Autodesk Inventor part; units mm, degrees
(part 2 of 3)
  line L685 (61.8832, -0.1639) -> (61.8305, -0.147) construction
  line L686 (61.936, -0.181) -> (61.8832, -0.1639) construction
  line L687 (61.9887, -0.1981) -> (61.936, -0.181) construction
  line L688 (62.0414, -0.2153) -> (61.9887, -0.1981) construction
  line L689 (62.379, -0.2964) -> (62.0414, -0.2153) construction
  line L690 (62.6505, -0.3259) -> (62.379, -0.2964) construction
  line L691 (62.891, -0.3235) -> (62.6505, -0.3259) construction
  line L692 (63.1221, -0.2997) -> (62.891, -0.3235) construction
  line L693 (63.3379, -0.2543) -> (63.1221, -0.2997) construction
  line L694 (63.5493, -0.1924) -> (63.3379, -0.2543) construction
  line L695 (63.7488, -0.1123) -> (63.5493, -0.1924) construction
  line L696 (63.9434, -0.0172) -> (63.7488, -0.1123) construction
  line L697 (64.1297, 0.0937) -> (63.9434, -0.0172) construction
  line L698 (64.3071, 0.22) -> (64.1297, 0.0937) construction
  line L699 (64.4815, 0.3591) -> (64.3071, 0.22) construction
  line L700 (64.6461, 0.5133) -> (64.4815, 0.3591) construction
  line L701 (64.8026, 0.6817) -> (64.6461, 0.5133) construction
  line L702 (64.9569, 0.8616) -> (64.8026, 0.6817) construction
  line L703 (65.103, 1.0551) -> (64.9569, 0.8616) construction
  line L704 (65.2411, 1.262) -> (65.103, 1.0551) construction
  line L705 (65.3711, 1.4821) -> (65.2411, 1.262) construction
  line L706 (65.4984, 1.7129) -> (65.3711, 1.4821) construction
  line L707 (65.62, 1.9556) -> (65.4984, 1.7129) construction
  line L708 (65.7341, 2.2106) -> (65.62, 1.9556) construction
  line L709 (65.906, 2.5468) -> (65.7341, 2.2106) construction
  line L710 (66.1036, 2.8725) -> (65.906, 2.5468) construction
  line L711 (66.3186, 3.1911) -> (66.1036, 2.8725) construction
  line L712 (66.548, 3.5036) -> (66.3186, 3.1911) construction
  line L713 (66.79, 3.8108) -> (66.548, 3.5036) construction
  line L714 (67.0435, 4.1129) -> (66.79, 3.8108) construction
  line L715 (67.3077, 4.4102) -> (67.0435, 4.1129) construction
  line L716 (67.5819, 4.7028) -> (67.3077, 4.4102) construction
  line L717 (67.8657, 4.991) -> (67.5819, 4.7028) construction
  line L718 (68.1585, 5.2747) -> (67.8657, 4.991) construction
  line L719 (68.4601, 5.5541) -> (68.1585, 5.2747) construction
  line L720 (68.7701, 5.8291) -> (68.4601, 5.5541) construction
  line L721 (69.0883, 6.0998) -> (68.7701, 5.8291) construction
  line L722 (69.4145, 6.3662) -> (69.0883, 6.0998) construction
  line L723 (69.7484, 6.6283) -> (69.4145, 6.3662) construction
  line L724 (70.0899, 6.886) -> (69.7484, 6.6283) construction
  line L725 (70.4388, 7.1393) -> (70.0899, 6.886) construction
  line L726 (70.7949, 7.3883) -> (70.4388, 7.1393) construction
  line L727 (71.1581, 7.6328) -> (70.7949, 7.3883) construction
  line L728 (71.5282, 7.8729) -> (71.1581, 7.6328) construction
  line L729 (71.855, 7.7148) -> (71.5282, 7.8729) construction
  line L730 (72.1807, 7.5544) -> (71.855, 7.7148) construction
  line L731 (72.5051, 7.3915) -> (72.1807, 7.5544) construction
  line L732 (72.8284, 7.2263) -> (72.5051, 7.3915) construction
  line L733 (73.1505, 7.0588) -> (72.8284, 7.2263) construction
  line L734 (73.4713, 6.8889) -> (73.1505, 7.0588) construction
  line L735 (73.7909, 6.7166) -> (73.4713, 6.8889) construction
  line L736 (74.1093, 6.5421) -> (73.7909, 6.7166) construction
  line L737 (74.4263, 6.3652) -> (74.1093, 6.5421) construction
  line L738 (74.7421, 6.186) -> (74.4263, 6.3652) construction
  line L739 (74.7421, 6.186) -> (69.921, -2.2381) construction
  arc A7 (69.921, -2.2381) -> (70.7543, -5.0163) centre (71.6568, -3.2315) ccw construction
  line L740 (70.7543, -5.0163) -> (83.2662, -11.3429) construction
  arc A8 (83.2662, -11.3429) -> (85.055, -11.351) centre (84.1687, -9.5581) ccw construction
  line L741 (85.055, -11.351) -> (116.4248, 4.1568) construction
  arc A9 (119.0371, 3.3744) -> (116.4248, 4.1568) centre (117.3112, 2.3639) ccw construction
  arc A10 (127.7114, -56.0453) -> (119.0371, 3.3744) centre (50, -37.0469) ccw construction
  arc A11 (43.6257, -5.6882) -> (19.6369, -47.1503) centre (50, -37.0469) ccw construction
  arc A12 (19.6369, -47.1503) -> (21.707, -48.5114) centre (21.5346, -46.5189) ccw construction
  line L742 (21.707, -48.5114) -> (35.3323, -47.3323) construction
  arc A13 (35.3323, -47.3323) -> (36.9058, -44.3641) centre (35.1599, -45.3397) ccw construction
  arc A14 (45.1164, -22.8641) -> (36.9058, -44.3641) centre (50, -37.0469) ccw construction
  arc A15 (45.1164, -22.8641) -> (46.4641, -20.9069) centre (44.4652, -20.9731) ccw construction
  line L743 (46.4641, -20.9069) -> (46.023, -7.5819) construction
  arc A16 (46.023, -7.5819) -> (43.6257, -5.6882) centre (44.0241, -7.6481) ccw construction
  arc A17 (57.4364, -24.02) -> (53.9351, -22.5722) centre (50, -37.0469) ccw construction
  arc A18 (57.4364, -24.02) -> (59.3143, -24.076) centre (58.4279, -22.2831) ccw construction
  line L744 (59.3143, -24.076) -> (73.5046, -17.061) construction
  arc A19 (73.5046, -17.061) -> (73.4583, -13.4531) centre (72.6182, -15.2681) ccw construction
  line L745 (73.4583, -13.4531) -> (57.1422, -5.9013) construction
  arc A20 (57.1422, -5.9013) -> (56.7223, -5.7609) centre (56.3021, -7.7163) ccw construction
  arc A21 (56.7223, -5.7609) -> (54.2866, -5.3353) centre (50, -37.0469) ccw construction
  arc A22 (54.2866, -5.3353) -> (52.0197, -7.3834) centre (54.0186, -7.3173) ccw construction
  line L746 (52.0197, -7.3834) -> (52.4608, -20.7084) construction
  arc A23 (52.4608, -20.7084) -> (53.9351, -22.5722) centre (54.4597, -20.6423) ccw construction
  arc A24 (123.9497, -39.7746) -> (120.0838, -13.2926) centre (50, -37.0469) ccw construction
  arc A25 (120.0838, -13.2926) -> (117.3033, -12.1418) centre (118.1896, -13.9346) ccw construction
  line L747 (117.3033, -12.1418) -> (79.5339, -30.8131) construction
  arc A26 (79.5339, -30.8131) -> (80.0834, -34.5775) centre (80.4202, -32.606) ccw construction
  line L748 (80.0834, -34.5775) -> (121.6143, -41.6723) construction
  arc A27 (121.6143, -41.6723) -> (123.9497, -39.7746) centre (121.9511, -39.7009) ccw construction
  circle A28 centre (80.4791, -21.9795) radius 1.2295 construction
  circle A29 centre (83.5145, -42.7723) radius 1.2295 construction
  circle A30 centre (98.3003, -45.2982) radius 1.2295 construction
  circle A31 centre (93.9257, -15.3321) radius 1.2295 construction
  circle A32 centre (50, -37.0469) radius 4 construction
  circle A33 centre (10, -122.0469) radius 1.6 construction
  line L749 (0, -87.0469) -> (20, -87.0469) construction
  line L750 (20, -87.0469) -> (20, -132.0469) construction
  line L751 (0, -132.0469) -> (20, -132.0469) construction
  line L752 (0, -87.0469) -> (0, -132.0469) construction
  circle A34 centre (10, -97.0469) radius 1.6 construction
  circle A35 centre (10, 47.9531) radius 1.6 construction
  line L753 (20, 12.9531) -> (0, 12.9531) construction
  line L754 (0, 57.9531) -> (0, 12.9531) construction
  line L755 (20, 57.9531) -> (0, 57.9531) construction
  line L756 (20, 57.9531) -> (20, 12.9531) construction
  circle A36 centre (10, 22.9531) radius 1.6 construction
  circle A37 centre (50, 24.7653) radius 4 construction
  line L757 (43.5439, 16.1699) -> (43.5808, 16.1423) construction
  line L758 (43.5071, 16.1977) -> (43.5439, 16.1699) construction
  line L759 (43.4704, 16.2256) -> (43.5071, 16.1977) construction
  line L760 (43.4338, 16.2537) -> (43.4704, 16.2256) construction
  line L761 (43.3973, 16.2819) -> (43.4338, 16.2537) construction
  line L762 (43.361, 16.3104) -> (43.3973, 16.2819) construction
  line L763 (43.1086, 16.4778) -> (43.361, 16.3104) construction
  line L764 (42.9044, 16.5756) -> (43.1086, 16.4778) construction
  line L765 (42.6758, 16.6731) -> (42.9044, 16.5756) construction
  line L766 (42.469, 16.7329) -> (42.6758, 16.6731) construction
  line L767 (42.2706, 16.7673) -> (42.469, 16.7329) construction
  line L768 (42.0769, 16.7804) -> (42.2706, 16.7673) construction
  line L769 (41.8782, 16.7823) -> (42.0769, 16.7804) construction
  line L770 (41.6755, 16.7728) -> (41.8782, 16.7823) construction
  line L771 (41.4782, 16.7425) -> (41.6755, 16.7728) construction
  line L772 (41.2858, 16.6918) -> (41.4782, 16.7425) construction
  line L773 (41.0896, 16.6304) -> (41.2858, 16.6918) construction
  line L774 (40.8915, 16.5563) -> (41.0896, 16.6304) construction
  line L775 (40.7008, 16.4595) -> (40.8915, 16.5563) construction
  line L776 (40.5115, 16.3468) -> (40.7008, 16.4595) construction
  line L777 (40.3175, 16.2253) -> (40.5115, 16.3468) construction
  line L778 (40.135, 16.077) -> (40.3175, 16.2253) construction
  line L779 (39.9489, 15.919) -> (40.135, 16.077) construction
  line L780 (39.767, 15.7432) -> (39.9489, 15.919) construction
  line L781 (39.5974, 15.5404) -> (39.767, 15.7432) construction
  line L782 (39.4169, 15.3374) -> (39.5974, 15.5404) construction
  line L783 (39.0835, 15.1378) -> (39.4169, 15.3374) construction
  line L784 (38.7191, 14.9743) -> (39.0835, 15.1378) construction
  line L785 (38.3325, 14.8381) -> (38.7191, 14.9743) construction
  line L786 (37.9275, 14.7263) -> (38.3325, 14.8381) construction
  line L787 (37.5062, 14.6376) -> (37.9275, 14.7263) construction
  line L788 (37.0703, 14.5712) -> (37.5062, 14.6376) construction
  line L789 (36.6212, 14.5267) -> (37.0703, 14.5712) construction
  line L790 (36.1601, 14.504) -> (36.6212, 14.5267) construction
  line L791 (35.6881, 14.503) -> (36.1601, 14.504) construction
  line L792 (35.2063, 14.5239) -> (35.6881, 14.503) construction
  line L793 (34.7154, 14.5666) -> (35.2063, 14.5239) construction
  line L794 (34.2166, 14.6313) -> (34.7154, 14.5666) construction
  line L795 (33.7106, 14.7183) -> (34.2166, 14.6313) construction
  line L796 (33.1984, 14.8275) -> (33.7106, 14.7183) construction
  line L797 (32.6809, 14.9593) -> (33.1984, 14.8275) construction
  line L798 (32.1588, 15.1139) -> (32.6809, 14.9593) construction
  line L799 (31.6332, 15.2912) -> (32.1588, 15.1139) construction
  line L800 (31.1048, 15.4916) -> (31.6332, 15.2912) construction
  line L801 (30.5745, 15.7152) -> (31.1048, 15.4916) construction
  line L802 (30.0432, 15.9621) -> (30.5745, 15.7152) construction
  line L803 (30.0213, 16.0118) -> (30.0432, 15.9621) construction
  line L804 (29.9996, 16.0616) -> (30.0213, 16.0118) construction
  line L805 (29.978, 16.1115) -> (29.9996, 16.0616) construction
  line L806 (29.9565, 16.1614) -> (29.978, 16.1115) construction
  line L807 (29.9351, 16.2113) -> (29.9565, 16.1614) construction
  line L808 (29.9138, 16.2613) -> (29.9351, 16.2113) construction
  line L809 (29.8927, 16.3114) -> (29.9138, 16.2613) construction
  line L810 (29.8717, 16.3615) -> (29.8927, 16.3114) construction
  line L811 (29.8509, 16.4117) -> (29.8717, 16.3615) construction
  line L812 (29.8301, 16.4619) -> (29.8509, 16.4117) construction
  line L813 (30.0199, 17.0162) -> (29.8301, 16.4619) construction
  line L814 (30.2257, 17.5536) -> (30.0199, 17.0162) construction
  line L815 (30.447, 18.0736) -> (30.2257, 17.5536) construction
  line L816 (30.683, 18.5756) -> (30.447, 18.0736) construction
  line L817 (30.933, 19.0593) -> (30.683, 18.5756) construction
  line L818 (31.1963, 19.524) -> (30.933, 19.0593) construction
  line L819 (31.4721, 19.9692) -> (31.1963, 19.524) construction
  line L820 (31.7597, 20.3944) -> (31.4721, 19.9692) construction
  line L821 (32.0584, 20.7992) -> (31.7597, 20.3944) construction
  line L822 (32.3674, 21.1829) -> (32.0584, 20.7992) construction
  line L823 (32.6861, 21.545) -> (32.3674, 21.1829) construction
  line L824 (33.0136, 21.8849) -> (32.6861, 21.545) construction
  line L825 (33.3492, 22.2018) -> (33.0136, 21.8849) construction
  line L826 (33.6922, 22.495) -> (33.3492, 22.2018) construction
  line L827 (34.0419, 22.7635) -> (33.6922, 22.495) construction
  line L828 (34.3977, 23.0061) -> (34.0419, 22.7635) construction
  line L829 (34.7588, 23.2209) -> (34.3977, 23.0061) construction
  line L830 (35.1247, 23.4055) -> (34.7588, 23.2209) construction
  line L831 (35.495, 23.5553) -> (35.1247, 23.4055) construction
  line L832 (35.8699, 23.6576) -> (35.495, 23.5553) construction
  line L833 (36.1413, 23.6472) -> (35.8699, 23.6576) construction
  line L834 (36.405, 23.6292) -> (36.1413, 23.6472) construction
  line L835 (36.6579, 23.6387) -> (36.405, 23.6292) construction
  line L836 (36.9007, 23.6635) -> (36.6579, 23.6387) construction
  line L837 (37.1341, 23.6926) -> (36.9007, 23.6635) construction
  line L838 (37.3561, 23.7483) -> (37.1341, 23.6926) construction
  line L839 (37.5685, 23.8069) -> (37.3561, 23.7483) construction
  line L840 (37.7703, 23.8775) -> (37.5685, 23.8069) construction
  line L841 (37.9609, 23.9691) -> (37.7703, 23.8775) construction
  line L842 (38.1412, 24.0682) -> (37.9609, 23.9691) construction
  line L843 (38.3109, 24.1719) -> (38.1412, 24.0682) construction
  line L844 (38.4694, 24.2932) -> (38.3109, 24.1719) construction
  line L845 (38.6166, 24.433) -> (38.4694, 24.2932) construction
  line L846 (38.7528, 24.5776) -> (38.6166, 24.433) construction
  line L847 (38.8775, 24.7264) -> (38.7528, 24.5776) construction
  line L848 (38.9901, 24.8934) -> (38.8775, 24.7264) construction
  line L849 (39.0901, 25.084) -> (38.9901, 24.8934) construction
  line L850 (39.178, 25.3165) -> (39.0901, 25.084) construction
  line L851 (39.2489, 25.5315) -> (39.178, 25.3165) construction
  line L852 (39.3028, 25.8295) -> (39.2489, 25.5315) construction
  line L853 (39.3075, 25.8754) -> (39.3028, 25.8295) construction
  line L854 (39.3123, 25.9213) -> (39.3075, 25.8754) construction
  line L855 (39.3174, 25.9671) -> (39.3123, 25.9213) construction
  line L856 (39.3226, 26.013) -> (39.3174, 25.9671) construction
  line L857 (39.3281, 26.0588) -> (39.3226, 26.013) construction
  line L858 (39.3337, 26.1045) -> (39.3281, 26.0588) construction
  line L859 (39.3396, 26.1503) -> (39.3337, 26.1045) construction
  line L860 (39.3456, 26.196) -> (39.3396, 26.1503) construction
  line L861 (39.3519, 26.2417) -> (39.3456, 26.196) construction
  line L862 (39.3583, 26.2874) -> (39.3519, 26.2417) construction
  line L863 (39.3772, 26.5897) -> (39.3583, 26.2874) construction
  line L864 (39.3597, 26.8154) -> (39.3772, 26.5897) construction
  line L865 (39.3299, 27.0621) -> (39.3597, 26.8154) construction
  line L866 (39.2783, 27.2712) -> (39.3299, 27.0621) construction
  line L867 (39.2089, 27.4602) -> (39.2783, 27.2712) construction
  line L868 (39.1234, 27.6345) -> (39.2089, 27.4602) construction
  line L869 (39.0256, 27.8074) -> (39.1234, 27.6345) construction
  line L870 (38.9161, 27.9783) -> (39.0256, 27.8074) construction
  line L871 (38.7911, 28.134) -> (38.9161, 27.9783) construction
  line L872 (38.6511, 28.2752) -> (38.7911, 28.134) construction
  line L873 (38.4997, 28.4145) -> (38.6511, 28.2752) construction
  line L874 (38.3366, 28.549) -> (38.4997, 28.4145) construction
  line L875 (38.1574, 28.6658) -> (38.3366, 28.549) construction
  line L876 (37.9652, 28.7734) -> (38.1574, 28.6658) construction
  line L877 (37.7629, 28.8805) -> (37.9652, 28.7734) construction
  line L878 (37.5432, 28.9645) -> (37.7629, 28.8805) construction
  line L879 (37.3134, 29.0466) -> (37.5432, 28.9645) construction
  line L880 (37.0701, 29.1163) -> (37.3134, 29.0466) construction
  line L881 (36.8097, 29.1618) -> (37.0701, 29.1163) construction
  line L882 (36.5437, 29.2166) -> (36.8097, 29.1618) construction
  line L883 (36.2041, 29.4055) -> (36.5437, 29.2166) construction
  line L884 (35.8803, 29.6394) -> (36.2041, 29.4055) construction
  line L885 (35.569, 29.906) -> (35.8803, 29.6394) construction
  line L886 (35.2697, 30.2009) -> (35.569, 29.906) construction
  line L887 (34.9822, 30.5214) -> (35.2697, 30.2009) construction
  line L888 (34.7068, 30.8657) -> (34.9822, 30.5214) construction
  line L889 (34.4437, 31.2324) -> (34.7068, 30.8657) construction
  line L890 (34.1935, 31.6203) -> (34.4437, 31.2324) construction
  line L891 (33.9567, 32.0286) -> (34.1935, 31.6203) construction
  line L892 (33.7338, 32.4563) -> (33.9567, 32.0286) construction
  line L893 (33.5254, 32.9028) -> (33.7338, 32.4563) construction
  line L894 (33.332, 33.3671) -> (33.5254, 32.9028) construction
  line L895 (33.1543, 33.8488) -> (33.332, 33.3671) construction
  line L896 (32.9929, 34.347) -> (33.1543, 33.8488) construction
  line L897 (32.8482, 34.8611) -> (32.9929, 34.347) construction
  line L898 (32.721, 35.3905) -> (32.8482, 34.8611) construction
  line L899 (32.6118, 35.9344) -> (32.721, 35.3905) construction
  line L900 (32.5212, 36.4922) -> (32.6118, 35.9344) construction
  line L901 (32.4496, 37.0632) -> (32.5212, 36.4922) construction
  line L902 (32.3978, 37.6468) -> (32.4496, 37.0632) construction
  line L903 (32.4299, 37.6906) -> (32.3978, 37.6468) construction
  line L904 (32.4622, 37.7343) -> (32.4299, 37.6906) construction
  line L905 (32.4945, 37.778) -> (32.4622, 37.7343) construction
  line L906 (32.527, 37.8215) -> (32.4945, 37.778) construction
  line L907 (32.5596, 37.865) -> (32.527, 37.8215) construction
  line L908 (32.5923, 37.9084) -> (32.5596, 37.865) construction
  line L909 (32.6251, 37.9518) -> (32.5923, 37.9084) construction
  line L910 (32.658, 37.995) -> (32.6251, 37.9518) construction
  line L911 (32.691, 38.0382) -> (32.658, 37.995) construction
  line L912 (32.7241, 38.0812) -> (32.691, 38.0382) construction
  line L913 (33.299, 38.194) -> (32.7241, 38.0812) construction
  line L914 (33.8673, 38.2844) -> (33.299, 38.194) construction
  line L915 (34.4283, 38.3528) -> (33.8673, 38.2844) construction
  line L916 (34.9811, 38.3995) -> (34.4283, 38.3528) construction
  line L917 (35.525, 38.4248) -> (34.9811, 38.3995) construction
  line L918 (36.059, 38.4291) -> (35.525, 38.4248) construction
  line L919 (36.5825, 38.4129) -> (36.059, 38.4291) construction
  line L920 (37.0946, 38.3764) -> (36.5825, 38.4129) construction
  line L921 (37.5944, 38.3201) -> (37.0946, 38.3764) construction
  line L922 (38.0813, 38.2443) -> (37.5944, 38.3201) construction
  line L923 (38.5542, 38.1494) -> (38.0813, 38.2443) construction
  line L924 (39.0122, 38.0358) -> (38.5542, 38.1494) construction
  line L925 (39.4545, 37.9036) -> (39.0122, 38.0358) construction
  line L926 (39.88, 37.7531) -> (39.4545, 37.9036) construction
  line L927 (40.2874, 37.5845) -> (39.88, 37.7531) construction
  line L928 (40.6753, 37.3977) -> (40.2874, 37.5845) construction
  line L929 (41.042, 37.1924) -> (40.6753, 37.3977) construction
  line L930 (41.3848, 36.9678) -> (41.042, 37.1924) construction
  line L931 (41.6996, 36.722) -> (41.3848, 36.9678) construction
  line L932 (41.9756, 36.4484) -> (41.6996, 36.722) construction
  line L933 (42.1024, 36.2082) -> (41.9756, 36.4484) construction
  line L934 (42.2186, 35.9708) -> (42.1024, 36.2082) construction
  line L935 (42.3533, 35.7566) -> (42.2186, 35.9708) construction
  line L936 (42.4962, 35.5588) -> (42.3533, 35.7566) construction
  line L937 (42.6381, 35.3711) -> (42.4962, 35.5588) construction
  line L938 (42.7974, 35.2068) -> (42.6381, 35.3711) construction
  line L939 (42.9543, 35.0521) -> (42.7974, 35.2068) construction
  line L940 (43.1163, 34.9126) -> (42.9543, 35.0521) construction
  line L941 (43.291, 34.7933) -> (43.1163, 34.9126) construction
  line L942 (43.4669, 34.6868) -> (43.291, 34.7933) construction
  line L943 (43.6416, 34.5916) -> (43.4669, 34.6868) construction
  line L944 (43.8259, 34.515) -> (43.6416, 34.5916) construction
  line L945 (44.0205, 34.4574) -> (43.8259, 34.515) construction
  line L946 (44.2138, 34.4117) -> (44.0205, 34.4574) construction
  line L947 (44.4051, 34.3782) -> (44.2138, 34.4117) construction
  line L948 (44.606, 34.3642) -> (44.4051, 34.3782) construction
  line L949 (44.8211, 34.3729) -> (44.606, 34.3642) construction
  line L950 (45.0664, 34.413) -> (44.8211, 34.3729) construction
  line L951 (45.288, 34.4591) -> (45.0664, 34.413) construction
  line L952 (45.5731, 34.5615) -> (45.288, 34.4591) construction
  line L953 (45.6151, 34.5804) -> (45.5731, 34.5615) construction
  line L954 (45.6573, 34.5991) -> (45.6151, 34.5804) construction
  line L955 (45.6995, 34.6176) -> (45.6573, 34.5991) construction
  line L956 (45.7418, 34.636) -> (45.6995, 34.6176) construction
  line L957 (45.7842, 34.6542) -> (45.7418, 34.636) construction
  line L958 (45.8267, 34.6722) -> (45.7842, 34.6542) construction
  line L959 (45.8692, 34.69) -> (45.8267, 34.6722) construction
  line L960 (45.9119, 34.7076) -> (45.8692, 34.69) construction
  line L961 (45.9546, 34.725) -> (45.9119, 34.7076) construction
  line L962 (45.9973, 34.7423) -> (45.9546, 34.725) construction
  line L963 (46.2685, 34.8771) -> (45.9973, 34.7423) construction
  line L964 (46.4553, 35.0051) -> (46.2685, 34.8771) construction
  line L965 (46.6541, 35.1543) -> (46.4553, 35.0051) construction
  line L966 (46.8093, 35.3035) -> (46.6541, 35.1543) construction
  line L967 (46.9383, 35.4581) -> (46.8093, 35.3035) construction
  line L968 (47.0465, 35.6193) -> (46.9383, 35.4581) construction
  line L969 (47.1474, 35.7905) -> (47.0465, 35.6193) construction
  line L970 (47.2406, 35.9708) -> (47.1474, 35.7905) construction
  line L971 (47.3129, 36.1568) -> (47.2406, 35.9708) construction
  line L972 (47.3652, 36.3487) -> (47.3129, 36.1568) construction
  line L973 (47.4102, 36.5494) -> (47.3652, 36.3487) construction
  line L974 (47.4451, 36.758) -> (47.4102, 36.5494) construction
  line L975 (47.4566, 36.9715) -> (47.4451, 36.758) construction
  line L976 (47.4537, 37.1918) -> (47.4566, 36.9715) construction
  line L977 (47.4454, 37.4206) -> (47.4537, 37.1918) construction
  line L978 (47.4082, 37.6528) -> (47.4454, 37.4206) construction
  line L979 (47.3644, 37.8929) -> (47.4082, 37.6528) construction
  line L980 (47.3031, 38.1384) -> (47.3644, 37.8929) construction
  line L981 (47.2124, 38.3867) -> (47.3031, 38.1384) construction
  line L982 (47.1268, 38.6444) -> (47.2124, 38.3867) construction
  line L983 (47.1206, 39.033) -> (47.1268, 38.6444) construction
  line L984 (47.1612, 39.4304) -> (47.1206, 39.033) construction
  line L985 (47.2365, 39.8332) -> (47.1612, 39.4304) construction
  line L986 (47.3422, 40.2399) -> (47.2365, 39.8332) construction
  line L987 (47.4761, 40.6491) -> (47.3422, 40.2399) construction
  line L988 (47.6365, 41.0598) -> (47.4761, 40.6491) construction
  line L989 (47.8225, 41.471) -> (47.6365, 41.0598) construction
  line L990 (48.0334, 41.8816) -> (47.8225, 41.471) construction
  line L991 (48.2686, 42.2908) -> (48.0334, 41.8816) construction
  line L992 (48.5275, 42.6977) -> (48.2686, 42.2908) construction
  line L993 (48.8099, 43.1015) -> (48.5275, 42.6977) construction
  line L994 (49.1154, 43.5011) -> (48.8099, 43.1015) construction
  line L995 (49.4437, 43.8958) -> (49.1154, 43.5011) construction
  line L996 (49.7944, 44.2848) -> (49.4437, 43.8958) construction
  line L997 (50.1674, 44.6671) -> (49.7944, 44.2848) construction
  line L998 (50.5622, 45.0419) -> (50.1674, 44.6671) construction
  line L999 (50.9787, 45.4085) -> (50.5622, 45.0419) construction
  line L1000 (51.4164, 45.7659) -> (50.9787, 45.4085) construction
  line L1001 (51.8752, 46.1133) -> (51.4164, 45.7659) construction
  line L1002 (52.3546, 46.45) -> (51.8752, 46.1133) construction
  line L1003 (52.4086, 46.4441) -> (52.3546, 46.45) construction
  line L1004 (52.4626, 46.438) -> (52.4086, 46.4441) construction
  line L1005 (52.5166, 46.4318) -> (52.4626, 46.438) construction
  line L1006 (52.5705, 46.4255) -> (52.5166, 46.4318) construction
  line L1007 (52.6245, 46.419) -> (52.5705, 46.4255) construction
  line L1008 (52.6784, 46.4124) -> (52.6245, 46.419) construction
  line L1009 (52.7324, 46.4056) -> (52.6784, 46.4124) construction
  line L1010 (52.7863, 46.3988) -> (52.7324, 46.4056) construction
  line L1011 (52.8401, 46.3918) -> (52.7863, 46.3988) construction
  line L1012 (52.894, 46.3846) -> (52.8401, 46.3918) construction
  line L1013 (53.2791, 45.9432) -> (52.894, 46.3846) construction
  line L1014 (53.6416, 45.4962) -> (53.2791, 45.9432) construction
  line L1015 (53.9813, 45.0445) -> (53.6416, 45.4962) construction
  line L1016 (54.2981, 44.5891) -> (53.9813, 45.0445) construction
  line L1017 (54.592, 44.1308) -> (54.2981, 44.5891) construction
  line L1018 (54.8628, 43.6705) -> (54.592, 44.1308) construction
  line L1019 (55.1104, 43.209) -> (54.8628, 43.6705) construction
  line L1020 (55.3349, 42.7473) -> (55.1104, 43.209) construction
  line L1021 (55.5361, 42.2862) -> (55.3349, 42.7473) construction
  line L1022 (55.7138, 41.8267) -> (55.5361, 42.2862) construction
  line L1023 (55.8681, 41.3697) -> (55.7138, 41.8267) construction
  line L1024 (55.9987, 40.9162) -> (55.8681, 41.3697) construction
  line L1025 (56.1054, 40.4671) -> (55.9987, 40.9162) construction
  line L1026 (56.1878, 40.0234) -> (56.1054, 40.4671) construction
  line L1027 (56.2455, 39.5863) -> (56.1878, 40.0234) construction
  line L1028 (56.2776, 39.1569) -> (56.2455, 39.5863) construction
  line L1029 (56.2832, 38.7367) -> (56.2776, 39.1569) construction
  line L1030 (56.26, 38.3276) -> (56.2832, 38.7367) construction
  line L1031 (56.2046, 37.932) -> (56.26, 38.3276) construction
  line L1032 (56.1057, 37.5562) -> (56.2046, 37.932) construction
  line L1033 (55.961, 37.3263) -> (56.1057, 37.5562) construction
  line L1034 (55.8136, 37.1069) -> (55.961, 37.3263) construction
  line L1035 (55.6954, 36.8832) -> (55.8136, 37.1069) construction
  line L1036 (55.5955, 36.6605) -> (55.6954, 36.8832) construction
  line L1037 (55.504, 36.4438) -> (55.5955, 36.6605) construction
  line L1038 (55.4413, 36.2237) -> (55.504, 36.4438) construction
  line L1039 (55.3858, 36.0105) -> (55.4413, 36.2237) construction
  line L1040 (55.3459, 35.8004) -> (55.3858, 36.0105) construction
  line L1041 (55.33, 35.5895) -> (55.3459, 35.8004) construction
  line L1042 (55.3257, 35.3839) -> (55.33, 35.5895) construction
  line L1043 (55.3307, 35.185) -> (55.3257, 35.3839) construction
  line L1044 (55.3565, 34.9871) -> (55.3307, 35.185) construction
  line L1045 (55.4039, 34.7897) -> (55.3565, 34.9871) construction
  line L1046 (55.461, 34.5995) -> (55.4039, 34.7897) construction
  line L1047 (55.5276, 34.4171) -> (55.461, 34.5995) construction
  line L1048 (55.6159, 34.2361) -> (55.5276, 34.4171) construction
  line L1049 (55.731, 34.0541) -> (55.6159, 34.2361) construction
  line L1050 (55.8883, 33.8618) -> (55.731, 34.0541) construction
  line L1051 (56.0391, 33.6929) -> (55.8883, 33.8618) construction
  line L1052 (56.2703, 33.4972) -> (56.0391, 33.6929) construction
  line L1053 (56.3077, 33.4702) -> (56.2703, 33.4972) construction
  line L1054 (56.345, 33.4431) -> (56.3077, 33.4702) construction
  line L1055 (56.3821, 33.4158) -> (56.345, 33.4431) construction
  line L1056 (56.4192, 33.3883) -> (56.3821, 33.4158) construction
  line L1057 (56.4561, 33.3607) -> (56.4192, 33.3883) construction
  line L1058 (56.4929, 33.3329) -> (56.4561, 33.3607) construction
  line L1059 (56.5296, 33.305) -> (56.4929, 33.3329) construction
  line L1060 (56.5662, 33.2769) -> (56.5296, 33.305) construction
  line L1061 (56.6027, 33.2486) -> (56.5662, 33.2769) construction
  line L1062 (56.639, 33.2202) -> (56.6027, 33.2486) construction
  line L1063 (56.8914, 33.0528) -> (56.639, 33.2202) construction
  line L1064 (57.0956, 32.955) -> (56.8914, 33.0528) construction
  line L1065 (57.3242, 32.8575) -> (57.0956, 32.955) construction
  line L1066 (57.531, 32.7977) -> (57.3242, 32.8575) construction
  line L1067 (57.7294, 32.7632) -> (57.531, 32.7977) construction
  line L1068 (57.9231, 32.7501) -> (57.7294, 32.7632) construction
  line L1069 (58.1218, 32.7483) -> (57.9231, 32.7501) construction
  line L1070 (58.3245, 32.7578) -> (58.1218, 32.7483) construction
  line L1071 (58.5218, 32.7881) -> (58.3245, 32.7578) construction
  line L1072 (58.7142, 32.8388) -> (58.5218, 32.7881) construction
  line L1073 (58.9104, 32.9002) -> (58.7142, 32.8388) construction
  line L1074 (59.1085, 32.9742) -> (58.9104, 32.9002) construction
  line L1075 (59.2992, 33.071) -> (59.1085, 32.9742) construction
  line L1076 (59.4885, 33.1837) -> (59.2992, 33.071) construction
  line L1077 (59.6825, 33.3053) -> (59.4885, 33.1837) construction
  line L1078 (59.865, 33.4536) -> (59.6825, 33.3053) construction
  line L1079 (60.0511, 33.6116) -> (59.865, 33.4536) construction
  line L1080 (60.233, 33.7874) -> (60.0511, 33.6116) construction
  line L1081 (60.4026, 33.9901) -> (60.233, 33.7874) construction
  line L1082 (60.5831, 34.1932) -> (60.4026, 33.9901) construction
  line L1083 (60.9165, 34.3928) -> (60.5831, 34.1932) construction
  line L1084 (61.2809, 34.5563) -> (60.9165, 34.3928) construction
  line L1085 (61.6675, 34.6925) -> (61.2809, 34.5563) construction
  line L1086 (62.0725, 34.8043) -> (61.6675, 34.6925) construction
  line L1087 (62.4938, 34.893) -> (62.0725, 34.8043) construction
  line L1088 (62.9297, 34.9594) -> (62.4938, 34.893) construction
  line L1089 (63.3788, 35.0039) -> (62.9297, 34.9594) construction
  line L1090 (63.8399, 35.0266) -> (63.3788, 35.0039) construction
  line L1091 (64.3119, 35.0275) -> (63.8399, 35.0266) construction
  line L1092 (64.7937, 35.0067) -> (64.3119, 35.0275) construction
  line L1093 (65.2846, 34.964) -> (64.7937, 35.0067) construction
  line L1094 (65.7834, 34.8992) -> (65.2846, 34.964) construction
  line L1095 (66.2894, 34.8123) -> (65.7834, 34.8992) construction
  line L1096 (66.8016, 34.703) -> (66.2894, 34.8123) construction
  line L1097 (67.3191, 34.5712) -> (66.8016, 34.703) construction
  line L1098 (67.8412, 34.4167) -> (67.3191, 34.5712) construction
  line L1099 (68.3668, 34.2393) -> (67.8412, 34.4167) construction
  line L1100 (68.8952, 34.0389) -> (68.3668, 34.2393) construction
  line L1101 (69.4255, 33.8154) -> (68.8952, 34.0389) construction
  line L1102 (69.9568, 33.5685) -> (69.4255, 33.8154) construction
  line L1103 (69.9787, 33.5188) -> (69.9568, 33.5685) construction
  line L1104 (70.0004, 33.469) -> (69.9787, 33.5188) construction
  line L1105 (70.022, 33.4191) -> (70.0004, 33.469) construction
  line L1106 (70.0435, 33.3692) -> (70.022, 33.4191) construction
  line L1107 (70.0649, 33.3193) -> (70.0435, 33.3692) construction
  line L1108 (70.0862, 33.2692) -> (70.0649, 33.3193) construction
  line L1109 (70.1073, 33.2192) -> (70.0862, 33.2692) construction
  line L1110 (70.1283, 33.1691) -> (70.1073, 33.2192) construction
  line L1111 (70.1491, 33.1189) -> (70.1283, 33.1691) construction
  line L1112 (70.1699, 33.0687) -> (70.1491, 33.1189) construction
  line L1113 (69.9801, 32.5144) -> (70.1699, 33.0687) construction
  line L1114 (69.7743, 31.977) -> (69.9801, 32.5144) construction
  line L1115 (69.553, 31.457) -> (69.7743, 31.977) construction
  line L1116 (69.317, 30.9549) -> (69.553, 31.457) construction
  line L1117 (69.067, 30.4713) -> (69.317, 30.9549) construction
  line L1118 (68.8037, 30.0066) -> (69.067, 30.4713) construction
  line L1119 (68.5279, 29.5614) -> (68.8037, 30.0066) construction
  line L1120 (68.2403, 29.1361) -> (68.5279, 29.5614) construction
  line L1121 (67.9416, 28.7314) -> (68.2403, 29.1361) construction
  line L1122 (67.6326, 28.3477) -> (67.9416, 28.7314) construction
  line L1123 (67.3139, 27.9856) -> (67.6326, 28.3477) construction
  line L1124 (66.9864, 27.6457) -> (67.3139, 27.9856) construction
  line L1125 (66.6508, 27.3288) -> (66.9864, 27.6457) construction
  line L1126 (66.3078, 27.0356) -> (66.6508, 27.3288) construction
  line L1127 (65.9581, 26.767) -> (66.3078, 27.0356) construction
  line L1128 (65.6023, 26.5245) -> (65.9581, 26.767) construction
  line L1129 (65.2412, 26.3096) -> (65.6023, 26.5245) construction
  line L1130 (64.8753, 26.1251) -> (65.2412, 26.3096) construction
  line L1131 (64.505, 25.9753) -> (64.8753, 26.1251) construction
  line L1132 (64.1301, 25.873) -> (64.505, 25.9753) construction
  line L1133 (63.8587, 25.8834) -> (64.1301, 25.873) construction
  line L1134 (63.595, 25.9014) -> (63.8587, 25.8834) construction
  line L1135 (63.3421, 25.8918) -> (63.595, 25.9014) construction
  line L1136 (63.0993, 25.867) -> (63.3421, 25.8918) construction
  line L1137 (62.8659, 25.838) -> (63.0993, 25.867) construction
  line L1138 (62.6439, 25.7822) -> (62.8659, 25.838) construction
  line L1139 (62.4315, 25.7237) -> (62.6439, 25.7822) construction
  line L1140 (62.2297, 25.6531) -> (62.4315, 25.7237) construction
  line L1141 (62.0391, 25.5615) -> (62.2297, 25.6531) construction
  line L1142 (61.8588, 25.4624) -> (62.0391, 25.5615) construction
  line L1143 (61.6891, 25.3587) -> (61.8588, 25.4624) construction
  line L1144 (61.5306, 25.2373) -> (61.6891, 25.3587) construction
  line L1145 (61.3834, 25.0976) -> (61.5306, 25.2373) construction
  line L1146 (61.2472, 24.953) -> (61.3834, 25.0976) construction
  line L1147 (61.1225, 24.8042) -> (61.2472, 24.953) construction
  line L1148 (61.0099, 24.6372) -> (61.1225, 24.8042) construction
  line L1149 (60.9099, 24.4466) -> (61.0099, 24.6372) construction
  line L1150 (60.822, 24.2141) -> (60.9099, 24.4466) construction
  line L1151 (60.7511, 23.9991) -> (60.822, 24.2141) construction
  line L1152 (60.6972, 23.701) -> (60.7511, 23.9991) construction
  line L1153 (60.6925, 23.6551) -> (60.6972, 23.701) construction
  line L1154 (60.6877, 23.6093) -> (60.6925, 23.6551) construction
  line L1155 (60.6826, 23.5634) -> (60.6877, 23.6093) construction
  line L1156 (60.6774, 23.5176) -> (60.6826, 23.5634) construction
  line L1157 (60.6719, 23.4718) -> (60.6774, 23.5176) construction
  line L1158 (60.6663, 23.426) -> (60.6719, 23.4718) construction
  line L1159 (60.6604, 23.3803) -> (60.6663, 23.426) construction
  line L1160 (60.6544, 23.3346) -> (60.6604, 23.3803) construction
  line L1161 (60.6481, 23.2889) -> (60.6544, 23.3346) construction
  line L1162 (60.6417, 23.2432) -> (60.6481, 23.2889) construction
  line L1163 (60.6228, 22.9409) -> (60.6417, 23.2432) construction
  line L1164 (60.6403, 22.7152) -> (60.6228, 22.9409) construction
  line L1165 (60.6701, 22.4685) -> (60.6403, 22.7152) construction
  line L1166 (60.7217, 22.2594) -> (60.6701, 22.4685) construction
  line L1167 (60.7911, 22.0704) -> (60.7217, 22.2594) construction
  line L1168 (60.8766, 21.8961) -> (60.7911, 22.0704) construction
  line L1169 (60.9744, 21.7231) -> (60.8766, 21.8961) construction
  line L1170 (61.0839, 21.5523) -> (60.9744, 21.7231) construction
  line L1171 (61.2089, 21.3966) -> (61.0839, 21.5523) construction
  line L1172 (61.3489, 21.2553) -> (61.2089, 21.3966) construction
  line L1173 (61.5003, 21.1161) -> (61.3489, 21.2553) construction
  line L1174 (61.6634, 20.9815) -> (61.5003, 21.1161) construction
  line L1175 (61.8426, 20.8648) -> (61.6634, 20.9815) construction
  line L1176 (62.0348, 20.7572) -> (61.8426, 20.8648) construction
  line L1177 (62.2371, 20.65) -> (62.0348, 20.7572) construction
  line L1178 (62.4568, 20.5661) -> (62.2371, 20.65) construction
  line L1179 (62.6866, 20.484) -> (62.4568, 20.5661) construction
  line L1180 (62.9299, 20.4143) -> (62.6866, 20.484) construction
  line L1181 (63.1903, 20.3688) -> (62.9299, 20.4143) construction
  line L1182 (63.4563, 20.314) -> (63.1903, 20.3688) construction
  line L1183 (63.7959, 20.1251) -> (63.4563, 20.314) construction
  line L1184 (64.1197, 19.8912) -> (63.7959, 20.1251) construction
  line L1185 (64.431, 19.6246) -> (64.1197, 19.8912) construction
  line L1186 (64.7303, 19.3297) -> (64.431, 19.6246) construction
  line L1187 (65.0178, 19.0092) -> (64.7303, 19.3297) construction
  line L1188 (65.2932, 18.6649) -> (65.0178, 19.0092) construction
  line L1189 (65.5563, 18.2982) -> (65.2932, 18.6649) construction
  line L1190 (65.8065, 17.9102) -> (65.5563, 18.2982) construction
  line L1191 (66.0433, 17.502) -> (65.8065, 17.9102) construction
  line L1192 (66.2662, 17.0742) -> (66.0433, 17.502) construction
  line L1193 (66.4746, 16.6278) -> (66.2662, 17.0742) construction
  line L1194 (66.668, 16.1634) -> (66.4746, 16.6278) construction
  line L1195 (66.8457, 15.6818) -> (66.668, 16.1634) construction
  line L1196 (67.0071, 15.1836) -> (66.8457, 15.6818) construction
  line L1197 (67.1518, 14.6694) -> (67.0071, 15.1836) construction
  line L1198 (67.279, 14.1401) -> (67.1518, 14.6694) construction
  line L1199 (67.3882, 13.5962) -> (67.279, 14.1401) construction
  line L1200 (67.4788, 13.0383) -> (67.3882, 13.5962) construction
  line L1201 (67.5504, 12.4673) -> (67.4788, 13.0383) construction
  line L1202 (67.6022, 11.8838) -> (67.5504, 12.4673) construction
  line L1203 (67.5701, 11.84) -> (67.6022, 11.8838) construction
  line L1204 (67.5378, 11.7963) -> (67.5701, 11.84) construction
  line L1205 (67.5055, 11.7526) -> (67.5378, 11.7963) construction
  line L1206 (67.473, 11.709) -> (67.5055, 11.7526) construction
  line L1207 (67.4404, 11.6656) -> (67.473, 11.709) construction
  line L1208 (67.4077, 11.6221) -> (67.4404, 11.6656) construction
  line L1209 (67.3749, 11.5788) -> (67.4077, 11.6221) construction
  line L1210 (67.342, 11.5356) -> (67.3749, 11.5788) construction
  line L1211 (67.309, 11.4924) -> (67.342, 11.5356) construction
  line L1212 (67.2759, 11.4493) -> (67.309, 11.4924) construction
  line L1213 (66.701, 11.3365) -> (67.2759, 11.4493) construction
  line L1214 (66.1327, 11.2461) -> (66.701, 11.3365) construction
  line L1215 (65.5717, 11.1778) -> (66.1327, 11.2461) construction
  line L1216 (65.0189, 11.1311) -> (65.5717, 11.1778) construction
  line L1217 (64.475, 11.1058) -> (65.0189, 11.1311) construction
  line L1218 (63.941, 11.1014) -> (64.475, 11.1058) construction
  line L1219 (63.4175, 11.1177) -> (63.941, 11.1014) construction
  line L1220 (62.9054, 11.1541) -> (63.4175, 11.1177) construction
  line L1221 (62.4056, 11.2105) -> (62.9054, 11.1541) construction
  line L1222 (61.9187, 11.2862) -> (62.4056, 11.2105) construction
  line L1223 (61.4458, 11.3811) -> (61.9187, 11.2862) construction
  line L1224 (60.9878, 11.4948) -> (61.4458, 11.3811) construction
  line L1225 (60.5455, 11.627) -> (60.9878, 11.4948) construction
  line L1226 (60.12, 11.7775) -> (60.5455, 11.627) construction
  line L1227 (59.7126, 11.9461) -> (60.12, 11.7775) construction
  line L1228 (59.3247, 12.1329) -> (59.7126, 11.9461) construction
  line L1229 (58.958, 12.3382) -> (59.3247, 12.1329) construction
  line L1230 (58.6152, 12.5628) -> (58.958, 12.3382) construction
  line L1231 (58.3004, 12.8086) -> (58.6152, 12.5628) construction
  line L1232 (58.0244, 13.0821) -> (58.3004, 12.8086) construction
  line L1233 (57.8976, 13.3224) -> (58.0244, 13.0821) construction
  line L1234 (57.7814, 13.5598) -> (57.8976, 13.3224) construction
  line L1235 (57.6467, 13.774) -> (57.7814, 13.5598) construction
  line L1236 (57.5038, 13.9718) -> (57.6467, 13.774) construction
  line L1237 (57.3619, 14.1594) -> (57.5038, 13.9718) construction
  line L1238 (57.2026, 14.3238) -> (57.3619, 14.1594) construction
  line L1239 (57.0457, 14.4785) -> (57.2026, 14.3238) construction
  line L1240 (56.8837, 14.618) -> (57.0457, 14.4785) construction
  line L1241 (56.709, 14.7372) -> (56.8837, 14.618) construction
  line L1242 (56.5331, 14.8438) -> (56.709, 14.7372) construction
  line L1243 (56.3584, 14.9389) -> (56.5331, 14.8438) construction
  line L1244 (56.1741, 15.0155) -> (56.3584, 14.9389) construction
  line L1245 (55.9795, 15.0732) -> (56.1741, 15.0155) construction
  line L1246 (55.7862, 15.1188) -> (55.9795, 15.0732) construction
  line L1247 (55.5949, 15.1524) -> (55.7862, 15.1188) construction
  line L1248 (55.394, 15.1664) -> (55.5949, 15.1524) construction
  line L1249 (55.1789, 15.1577) -> (55.394, 15.1664) construction
  line L1250 (54.9336, 15.1176) -> (55.1789, 15.1577) construction
  line L1251 (54.712, 15.0715) -> (54.9336, 15.1176) construction
  line L1252 (54.4269, 14.9691) -> (54.712, 15.0715) construction
  line L1253 (54.3849, 14.9502) -> (54.4269, 14.9691) construction
  line L1254 (54.3427, 14.9315) -> (54.3849, 14.9502) construction
  line L1255 (54.3005, 14.913) -> (54.3427, 14.9315) construction
  line L1256 (54.2582, 14.8946) -> (54.3005, 14.913) construction
  line L1257 (54.2158, 14.8764) -> (54.2582, 14.8946) construction
  line L1258 (54.1733, 14.8584) -> (54.2158, 14.8764) construction
  line L1259 (54.1308, 14.8406) -> (54.1733, 14.8584) construction
  line L1260 (54.0881, 14.823) -> (54.1308, 14.8406) construction
  line L1261 (54.0454, 14.8055) -> (54.0881, 14.823) construction
  line L1262 (54.0027, 14.7883) -> (54.0454, 14.8055) construction
  line L1263 (53.7315, 14.6534) -> (54.0027, 14.7883) construction
  line L1264 (53.5447, 14.5255) -> (53.7315, 14.6534) construction
  line L1265 (53.3459, 14.3763) -> (53.5447, 14.5255) construction
  line L1266 (53.1907, 14.2271) -> (53.3459, 14.3763) construction
  line L1267 (53.0617, 14.0725) -> (53.1907, 14.2271) construction
  line L1268 (52.9535, 13.9112) -> (53.0617, 14.0725) construction
  line L1269 (52.8526, 13.7401) -> (52.9535, 13.9112) construction
  line L1270 (52.7594, 13.5598) -> (52.8526, 13.7401) construction
  line L1271 (52.6871, 13.3738) -> (52.7594, 13.5598) construction
  line L1272 (52.6348, 13.1818) -> (52.6871, 13.3738) construction
  line L1273 (52.5898, 12.9812) -> (52.6348, 13.1818) construction
  line L1274 (52.5549, 12.7726) -> (52.5898, 12.9812) construction
  line L1275 (52.5434, 12.559) -> (52.5549, 12.7726) construction
  line L1276 (52.5463, 12.3388) -> (52.5434, 12.559) construction
  line L1277 (52.5546, 12.11) -> (52.5463, 12.3388) construction
  line L1278 (52.5918, 11.8778) -> (52.5546, 12.11) construction
  line L1279 (52.6356, 11.6377) -> (52.5918, 11.8778) construction
  line L1280 (52.6969, 11.3922) -> (52.6356, 11.6377) construction
  line L1281 (52.7876, 11.1439) -> (52.6969, 11.3922) construction
  line L1282 (52.8732, 10.8861) -> (52.7876, 11.1439) construction
  line L1283 (52.8794, 10.4976) -> (52.8732, 10.8861) construction
  line L1284 (52.8388, 10.1002) -> (52.8794, 10.4976) construction
  line L1285 (52.7635, 9.6974) -> (52.8388, 10.1002) construction
  line L1286 (52.6578, 9.2907) -> (52.7635, 9.6974) construction
  line L1287 (52.5239, 8.8814) -> (52.6578, 9.2907) construction
  line L1288 (52.3635, 8.4707) -> (52.5239, 8.8814) construction
  line L1289 (52.1775, 8.0596) -> (52.3635, 8.4707) construction
  line L1290 (51.9666, 7.649) -> (52.1775, 8.0596) construction
  line L1291 (51.7314, 7.2397) -> (51.9666, 7.649) construction
  line L1292 (51.4725, 6.8328) -> (51.7314, 7.2397) construction
  line L1293 (51.1901, 6.4291) -> (51.4725, 6.8328) construction
  line L1294 (50.8846, 6.0295) -> (51.1901, 6.4291) construction
  line L1295 (50.5563, 5.6348) -> (50.8846, 6.0295) construction
  line L1296 (50.2056, 5.2458) -> (50.5563, 5.6348) construction
  line L1297 (49.8326, 4.8635) -> (50.2056, 5.2458) construction
  line L1298 (49.4378, 4.4887) -> (49.8326, 4.8635) construction
  line L1299 (49.0213, 4.1221) -> (49.4378, 4.4887) construction
  line L1300 (48.5836, 3.7647) -> (49.0213, 4.1221) construction
  line L1301 (48.1248, 3.4172) -> (48.5836, 3.7647) construction
  line L1302 (47.6454, 3.0806) -> (48.1248, 3.4172) construction
  line L1303 (47.5914, 3.0865) -> (47.6454, 3.0806) construction
  line L1304 (47.5374, 3.0926) -> (47.5914, 3.0865) construction
  line L1305 (47.4834, 3.0988) -> (47.5374, 3.0926) construction
  line L1306 (47.4295, 3.1051) -> (47.4834, 3.0988) construction
  line L1307 (47.3755, 3.1116) -> (47.4295, 3.1051) construction
  line L1308 (47.3216, 3.1182) -> (47.3755, 3.1116) construction
  line L1309 (47.2676, 3.1249) -> (47.3216, 3.1182) construction
  line L1310 (47.2137, 3.1318) -> (47.2676, 3.1249) construction
  line L1311 (47.1599, 3.1388) -> (47.2137, 3.1318) construction
  line L1312 (47.106, 3.146) -> (47.1599, 3.1388) construction
  line L1313 (46.7209, 3.5874) -> (47.106, 3.146) construction
  line L1314 (46.3584, 4.0344) -> (46.7209, 3.5874) construction
  line L1315 (46.0187, 4.486) -> (46.3584, 4.0344) construction
  line L1316 (45.7019, 4.9415) -> (46.0187, 4.486) construction
  line L1317 (45.408, 5.3998) -> (45.7019, 4.9415) construction
  line L1318 (45.1372, 5.8601) -> (45.408, 5.3998) construction
  line L1319 (44.8896, 6.3216) -> (45.1372, 5.8601) construction
  line L1320 (44.6651, 6.7833) -> (44.8896, 6.3216) construction
  line L1321 (44.4639, 7.2443) -> (44.6651, 6.7833) construction
  line L1322 (44.2862, 7.7038) -> (44.4639, 7.2443) construction
  line L1323 (44.1319, 8.1608) -> (44.2862, 7.7038) construction
  line L1324 (44.0013, 8.6144) -> (44.1319, 8.1608) construction
  line L1325 (43.8946, 9.0635) -> (44.0013, 8.6144) construction
  line L1326 (43.8122, 9.5072) -> (43.8946, 9.0635) construction
  line L1327 (43.7545, 9.9443) -> (43.8122, 9.5072) construction
  line L1328 (43.7224, 10.3737) -> (43.7545, 9.9443) construction
  line L1329 (43.7168, 10.7938) -> (43.7224, 10.3737) construction
  line L1330 (43.74, 11.203) -> (43.7168, 10.7938) construction
  line L1331 (43.7954, 11.5986) -> (43.74, 11.203) construction
  line L1332 (43.8943, 11.9744) -> (43.7954, 11.5986) construction
  line L1333 (44.039, 12.2043) -> (43.8943, 11.9744) construction
  line L1334 (44.1864, 12.4236) -> (44.039, 12.2043) construction
  line L1335 (44.3046, 12.6474) -> (44.1864, 12.4236) construction
  line L1336 (44.4045, 12.8701) -> (44.3046, 12.6474) construction
  line L1337 (44.496, 13.0868) -> (44.4045, 12.8701) construction
  line L1338 (44.5587, 13.3069) -> (44.496, 13.0868) construction
  line L1339 (44.6142, 13.5201) -> (44.5587, 13.3069) construction
  line L1340 (44.6541, 13.7302) -> (44.6142, 13.5201) construction
  line L1341 (44.67, 13.9411) -> (44.6541, 13.7302) construction
  line L1342 (44.6743, 14.1467) -> (44.67, 13.9411) construction
  line L1343 (44.6693, 14.3456) -> (44.6743, 14.1467) construction
  line L1344 (44.6435, 14.5435) -> (44.6693, 14.3456) construction
  line L1345 (44.5961, 14.7408) -> (44.6435, 14.5435) construction
  line L1346 (44.539, 14.9311) -> (44.5961, 14.7408) construction
  line L1347 (44.4724, 15.1135) -> (44.539, 14.9311) construction
  line L1348 (44.3841, 15.2944) -> (44.4724, 15.1135) construction
  line L1349 (44.269, 15.4764) -> (44.3841, 15.2944) construction
  line L1350 (44.1117, 15.6688) -> (44.269, 15.4764) construction
  line L1351 (43.9609, 15.8377) -> (44.1117, 15.6688) construction
  line L1352 (43.7297, 16.0334) -> (43.9609, 15.8377) construction
  line L1353 (43.6923, 16.0604) -> (43.7297, 16.0334) construction
  line L1354 (43.655, 16.0875) -> (43.6923, 16.0604) construction
  line L1355 (43.6179, 16.1148) -> (43.655, 16.0875) construction
  line L1356 (43.5808, 16.1423) -> (43.6179, 16.1148) construction
  circle A38 centre (50, 24.7653) radius 4 construction
  circle A39 centre (50, -37.0469) radius 4 construction
  circle A40 centre (72.5, 11.9531) radius 1.6 construction
  circle A41 centre (27.5, -71.0469) radius 1.6 construction
  circle A42 centre (27.5, 11.9531) radius 1.6 construction
  line L1357 (62.6183, 32.8757) -> (75.0237, 13.5752) construction
  arc A43 (75.4366, 11.3394) -> (75.0237, 13.5752) centre (72.5, 11.9531) ccw construction
  line L1358 (75.4366, 11.3394) -> (64.6828, -40.1155) construction
  arc A44 (59.5184, -48.64) -> (64.6828, -40.1155) centre (50, -37.0469) ccw construction
  line L1359 (59.5184, -48.64) -> (29.4037, -73.3655) construction
  arc A45 (24.5, -71.0469) -> (29.4037, -73.3655) centre (27.5, -71.0469) ccw construction
  line L1360 (24.5, -71.0469) -> (24.5, 11.9531) construction
  arc A46 (24.9763, 13.5752) -> (24.5, 11.9531) centre (27.5, 11.9531) ccw construction
  line L1361 (24.9763, 13.5752) -> (37.3817, 32.8757) construction
  arc A47 (62.6183, 32.8757) -> (37.3817, 32.8757) centre (50, 24.7653) ccw construction
  arc A48 (16.4732, -132.0469) -> (21.7155, -128.9655) centre (16.4732, -126.0469) ccw construction
  line L1362 (67.4743, -46.7756) -> (21.7155, -128.9655) construction
  arc A49 (67.4743, -46.7756) -> (69.7797, -40.007) centre (50, -37.0469) ccw construction
  line L1363 (77.4449, 11.2131) -> (69.7797, -40.007) construction
  arc A50 (77.4449, 11.2131) -> (77.2948, 13.3708) centre (72.5, 11.9531) ccw construction
  line L1364 (61.2948, 67.483) -> (77.2948, 13.3708) construction
  arc A51 (61.2948, 67.483) -> (58.5953, 70.6051) centre (56.5, 66.0653) ccw construction
  line L1365 (52.0953, 73.6051) -> (58.5953, 70.6051) construction
  arc A52 (52.0953, 73.6051) -> (47.9047, 73.6051) centre (50, 69.0653) ccw construction
  line L1366 (41.4047, 70.6051) -> (47.9047, 73.6051) construction
  arc A53 (41.4047, 70.6051) -> (40.9513, 70.3669) centre (43.5, 66.0653) ccw construction
  line L1367 (21.4144, 58.7912) -> (40.9513, 70.3669) construction
  arc A54 (18.3559, 57.9531) -> (21.4144, 58.7912) centre (18.3559, 63.9531) ccw construction
  line L1368 (6, 57.9531) -> (18.3559, 57.9531) construction
  arc A55 (6, 57.9531) -> (0, 51.9531) centre (6, 51.9531) ccw construction
  line L1369 (0, 51.9531) -> (0, 18.9531) construction
  arc A56 (0, 18.9531) -> (6, 12.9531) centre (6, 18.9531) ccw construction
  line L1370 (14, 12.9531) -> (6, 12.9531) construction
  arc A57 (20, 6.9531) -> (14, 12.9531) centre (14, 6.9531) ccw construction
  line L1371 (20, -81.0469) -> (20, 6.9531) construction
  arc A58 (14, -87.0469) -> (20, -81.0469) centre (14, -81.0469) ccw construction
  line L1372 (6, -87.0469) -> (14, -87.0469) construction
  arc A59 (6, -87.0469) -> (0, -93.0469) centre (6, -93.0469) ccw construction
  line L1373 (0, -93.0469) -> (0, -126.0469) construction
  arc A60 (0, -126.0469) -> (6, -132.0469) centre (6, -126.0469) ccw construction
  line L1374 (16.4732, -132.0469) -> (6, -132.0469) construction
  circle A61 centre (10, -122.0469) radius 1.6 construction
  circle A62 centre (10, 47.9531) radius 1.6 construction